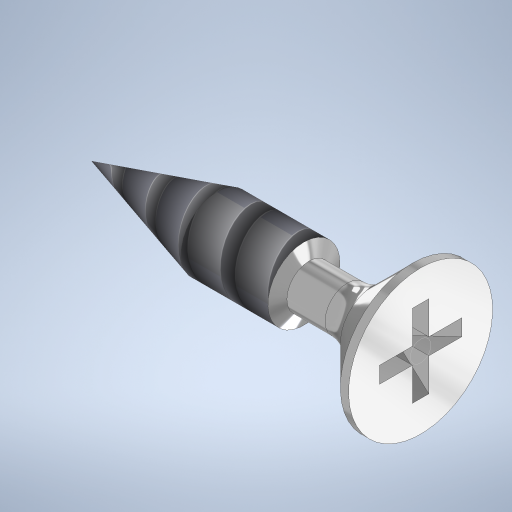
# Autodesk Inventor part: Wood screw Cross Recessed Flat Head M3.5x16 H
Saved by Autodesk Inventor 2024 (Build 280153000, 153)
## iProperties
Created: 2015-02-10
Part Number: Wood screw Cross Recessed Flat Head M3.5x16 H
Material: Steel
Document SubType Name: Modeling
Designer: SauliusD
Mass: 0.47398 g
Surface Area: 1.34781 cm^2
Volume: 0.0603796 cm^3
Density: 7.85 g/cm^3
Appearance: Plate
Description: Wood screw Cross Recessed Flat Head
Author: SauliusD
Autodesk Inventor part; units mm, degrees
ref_plane "YZ Plane" through (0, 0, 0) normal (1, 0, 0) x (0, 1, 0)
ref_plane "XZ Plane" through (0, 0, 0) normal (0, 1, 0) x (-1, 0, 0)
ref_plane "XY Plane" through (0, 0, 0) normal (0, 0, 1) x (1, 0, 0)
sketch "Sketch1" plane through (0, 0, 0) normal (0, 1, 0) x (-1, 0, 0)
  line L0 (0, 0) -> (0, 3.5)
  line L1 (0, 3.5) -> (0.4, 3.5)
  line L2 (0.4, 3.5) -> (2.825, 1.075)
  line L3 (2.825, 1.075) -> (5.425, 1.075)
  line L4 (5.425, 1.075) -> (5.6707, 1.75)
  line L5 (5.6707, 1.75) -> (9.897, 1.75)
  line L6 (9.897, 1.75) -> (16, 0)
  line L7 (16, 0) -> (0, 0)
  dimension "d0" = 7
  dimension "d1" = 45
  dimension "d2" = 16
  dimension "d3" = 2.6
  dimension "d4" = 110
  dimension "d5" = 2.15
  dimension "d6" = 3.5
  dimension "d7" = 0.4
  dimension "d8" = 16
  constraints: 16 end point, 3 parallel, 1 perpendicular, 1 vertical
  measures "d0" diameter of L1 L7
  measures "d1" angle of L0 L2
  measures "d2" angle of L7 L6
  measures "d3" distance of L2.end L3.end
  measures "d4" angle of L4 L3
  measures "d5" diameter of L3 L7
  measures "d6" diameter of L5 L7
  measures "d7" distance of L0.end L1.end
  measures "d8" distance of L6.end L0.start
revolve "Revolution1" add sketch "Sketch1" angle 360 about axis through (-16, 0, 0) along (1, 0, 0)
sketch "Sketch2" plane through (0, 0, 0) normal (0, 0, 1) x (1, 0, 0)
  line L0 (0, 3.5) -> (0, -3.5) projected
  line L1 (0, -2) -> (-1.76, -0.4)
  line L2 (-1.76, -0.4) -> (-1.76, 0.4)
  line L3 (-1.76, 0.4) -> (0, 2)
  line L4 (-2.112, 0) -> (0.352, 0) projected
  point P0 (0, 0)
  dimension "d10" = 4
  dimension "d11" = 1.76
  dimension "d12" = 0.8
  constraints: 6 end point, 2 point on line, 1 vertical, 1 other
  measures "d10" distance of L3.end L1.start
  measures "d11" distance between parallel lines of L0 L2
  measures "d12" distance of L1.end L2.end
extrude "Extrusion1" cut sketch "Sketch2" along normal mid plane 0.8
pattern_circular "Circular Pattern1" count 2 over 90 about axis through (-10, 0, 0) along (1, 0, 0) of "Extrusion1"
fillet "Fillet1" radius 1.8 1 edges at (-2.825, 0, -1.075)
thread "Thread1" size "R 3" standard "ISO Taper" full length
sketch "Sketch3" plane through (0, 0, 0) normal (1, 0, 0) x (0, 1, 0)
  circle A0 centre (0, 0) radius 0.5
  dimension "d21" = 1
  constraints: 1 centre point, 1 coincident
  measures "d21" diameter of A0
extrude "Extrusion2" add sketch "Sketch3" against normal blind 13 separate body
thread "Thread2" size "R 6" standard "ISO Taper" full length
equation "\"d10\" = M"
equation "\"d11\" = Q"
equation "\"d18\" = R"
equation "\"d19\" = L"
equation "\"d0\" = A_H"
equation "\"d3\" = a"
equation "\"d5\" = d"
equation "\"d6\" = D"
equation "\"d8\" = L"
equation "\"D\" = 3.5"
equation "\"a\" = 2.6"
equation "\"d\" = 2.15"
equation "\"P\" = 1.6"
equation "\"Q\" = 1.76"
equation "\"M\" = 4"
equation "\"A_H\" = 7"
equation "\"R\" = 1.8"
equation "\"L\" = 16"
body "Solid1"
